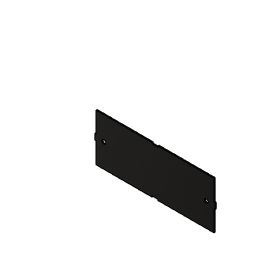
004_nixie_back_plate (Autodesk Fusion 360 design; units mm, degrees)
Autodesk Fusion 360 part; units mm, degrees
sketch "Sketch1" plane through (0, 0, -14) normal (0, 0, -1) x (-1, 0, 0)
  line L0 (-150, 118.5) -> (-150, 100) construction
  line L1 (-149, 100) -> (-149, 118.5) construction
  line L2 (-149, 118.5) -> (-150, 118.5) construction
  line L3 (-149, 72.5) -> (-149, 114.5) construction
  line L4 (-256, 98.75) -> (-256, 88.25) construction
  line L5 (-256, 110.75) -> (-256, 100.25) construction
  line L6 (-256, 86.75) -> (-256, 76.25) construction
  line L7 (-256, 114.5) -> (-256, 72.5) construction
  line L8 (-256, 72.5) -> (-256, 73.5) construction
  line L9 (-256, 73.5) -> (-256, 72.5) construction
  line L10 (-256, 91) -> (-256, 96) construction
  line L11 (-256, 114.5) -> (-256, 113.5) construction
  line L12 (-256, 113.5) -> (-256, 114.5) construction
  line L13 (-255, 98.75) -> (-255, 88.25) construction
  line L14 (-255, 110.75) -> (-255, 100.25) construction
  line L15 (-255, 86.75) -> (-255, 76.25) construction
  line L16 (-255, 72.5) -> (-255, 114.5) construction
  line L17 (-255, 114.5) -> (-255, 113.5) construction
  line L18 (-255, 113.5) -> (-255, 114.5) construction
  line L19 (-255, 96) -> (-255, 91) construction
  line L20 (-255, 72.5) -> (-255, 73.5) construction
  line L21 (-255, 73.5) -> (-255, 72.5) construction
  line L22 (-150, 114.5) -> (-150, 72.5) construction
  line L23 (-255, 114.5) -> (-150, 114.5)
  line L24 (-150, 114.5) -> (-150, 72.5)
  line L25 (-150, 72.5) -> (-255, 72.5)
  line L26 (-255, 72.5) -> (-255, 114.5)
  line L27 (-255, 96) -> (-256, 96)
  line L28 (-256, 96) -> (-256, 91)
  line L29 (-256, 91) -> (-255, 91)
  line L30 (-255, 91) -> (-255, 96)
  line L31 (-202.5, 114.5) -> (-202.5, 72.5) construction
  line L32 (-205, 114.5) -> (-200, 114.5)
  line L33 (-200, 114.5) -> (-200, 113.5)
  line L34 (-200, 113.5) -> (-205, 113.5)
  line L35 (-205, 113.5) -> (-205, 114.5)
  line L36 (-205, 72.5) -> (-200, 72.5)
  line L37 (-200, 72.5) -> (-200, 73.5)
  line L38 (-200, 73.5) -> (-205, 73.5)
  line L39 (-205, 73.5) -> (-205, 72.5)
  line L40 (-256, 72.5) -> (-256, 91)
  line L41 (-256, 96) -> (-256, 114.5)
  line L42 (-255, 114.5) -> (-255, 96)
  line L43 (-255, 91) -> (-255, 72.5)
  line L44 (-150, 72.5) -> (-149, 72.5)
  line L45 (-150, 96) -> (-150, 91)
  line L46 (-150, 91) -> (-149, 91)
  line L47 (-149, 91) -> (-149, 96)
  line L48 (-149, 96) -> (-150, 96)
  line L49 (-150, 114.5) -> (-150, 96)
  line L50 (-150, 96) -> (-149, 96)
  line L51 (-149, 96) -> (-149, 114.5)
  line L52 (-149, 114.5) -> (-150, 114.5)
  dimension "d456" = 5
  dimension "d457" = 1
  constraint horizontal L23
  constraint horizontal L25
  constraint vertical L26
  constraint coincident L16.end L17.start
  constraint horizontal L27
  constraint vertical L28
  constraint horizontal L29
  constraint vertical L30
  constraint coincident L10.start L28.end
  constraint coincident L19.start L27.start
  constraint midpoint L23 L31.start
  constraint midpoint L25 L31.end
  constraint horizontal L32
  constraint vertical L33
  constraint horizontal L34
  constraint vertical L35
  constraint coincident L23 L32.start
  constraint horizontal L36
  constraint vertical L37
  constraint horizontal L38
  constraint vertical L39
  constraint coincident L25 L36.start
  constraint symmetric L31 L33 L35
  constraint symmetric L31 L37 L39
  constraint equal L34 L38
  constraint equal L35 L39
  constraint collinear L0 L24
  constraint collinear L25 L44
  measures "d456" distance of L33.end L34.end
  measures "d457" distance of L32.start L34.end
extrude "Extrude1" add sketch "Sketch1" against normal blind 1 contours L23 L24 L25 L26 L30 L33 L34 L35 L37 L38 L39 L42 L43 L45 L49 | L26 L27 L28 L29 L30 | L24 L45 L46 L47 L48 L50
sketch "Sketch3" plane through (0, 0, -14) normal (0, 0, -1) x (-1, 0, 0)
  line L0 (-200, 114.5) -> (-200, 113.5)
  line L1 (-200, 113.5) -> (-205, 113.5)
  line L2 (-205, 113.5) -> (-205, 114.5)
  line L3 (-205, 114.5) -> (-255, 114.5)
  line L4 (-255, 114.5) -> (-255, 96)
  line L5 (-255, 96) -> (-256, 96)
  line L6 (-256, 96) -> (-256, 91)
  line L7 (-256, 91) -> (-255, 91)
  line L8 (-255, 91) -> (-255, 72.5)
  line L9 (-255, 72.5) -> (-205, 72.5)
  line L10 (-205, 72.5) -> (-205, 73.5)
  line L11 (-205, 73.5) -> (-200, 73.5)
  line L12 (-200, 73.5) -> (-200, 72.5)
  line L13 (-200, 72.5) -> (-150, 72.5)
  line L14 (-150, 72.5) -> (-150, 91)
  line L15 (-150, 96) -> (-150, 114.5)
  line L16 (-150, 114.5) -> (-200, 114.5)
  circle A0 centre (-248, 93.5) radius 2.5 construction
  circle A1 centre (-157, 93.5) radius 2.5 construction
  circle A2 centre (-248, 93.5) radius 2
  circle A3 centre (-157, 93.5) radius 2
  line L17 (-150, 91) -> (-149, 91)
  line L18 (-149, 91) -> (-149, 96)
  line L19 (-149, 96) -> (-150, 96)
  dimension "d745" = -0.5
  dimension "d746" = -0.5
hole "Hole1" at (248, 93.5, -14) at (157, 93.5, -14) direction (0, 0, 1) diameter 3.4 end up to surface (1 mm away)
equation "d746 = d745"
